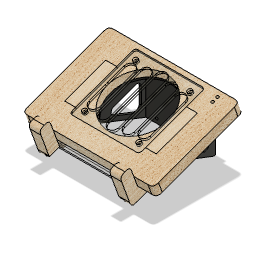
model_v2 (Autodesk Fusion 360 design; units mm, degrees)
Autodesk Fusion 360 part; units mm, degrees
note: some values were not read from the file. Set by a fixed rule: which face or edge a step refers to.
ref_plane "WorkPlane1" through (12.125, 0, 0) normal (0, -0.939693, -0.34202) x (1, 0, 0) in component "3dp"
sketch "Sketch1" plane through (12.125, 0, 0) normal (0, -0.939693, -0.34202) x (1, 0, 0) in component "3dp"
  line L0 (-87.125, 0) -> (62.875, 0)
  line L1 (62.875, 0) -> (62.875, 170)
  line L2 (62.875, 170) -> (-87.125, 170)
  line L3 (-87.125, 170) -> (-87.125, 0)
  line L4 (-12.125, 0) -> (-12.125, 170)
  line L5 (-87.125, 90) -> (62.875, 90) construction
  circle A0 centre (-12.125, 90) radius 70.05
  line L6 (-74.375, 27.75) -> (50.125, 27.75) construction
  line L7 (50.125, 27.75) -> (50.125, 152.25) construction
  line L8 (50.125, 152.25) -> (-74.375, 152.25) construction
  line L9 (-74.375, 152.25) -> (-74.375, 27.75) construction
  line L10 (-74.375, 27.75) -> (50.125, 152.25) construction
  line L11 (50.125, 27.75) -> (-74.375, 152.25) construction
  circle A1 centre (-74.375, 27.75) radius 2.25
  circle A2 centre (50.125, 27.75) radius 2.25
  circle A3 centre (50.125, 152.25) radius 2.25
  circle A4 centre (-74.375, 152.25) radius 2.25
  point P0 (-12.125, 90)
  point P1 (-12.125, 0)
  dimension "d2" = 150
  dimension "d3" = 170
  dimension "d4" = 90
  dimension "d5" = 140.1
  dimension "d6" = 124.5
  dimension "d7" = 124.5
  dimension "d8" = 4.5
  dimension "d9" = 4.5
  dimension "d10" = 4.5
  dimension "d11" = 4.5
  constraint horizontal L0
  constraint vertical L1
  constraint horizontal L2
  constraint vertical L3
  constraint midpoint L0 P1
  constraint midpoint L2 L4.end
  constraint coincident L3 L5.start
  constraint coincident L1 L5.end
  constraint perpendicular L1 L5
  constraint midpoint L5 P0
  constraint horizontal L6
  constraint perpendicular L6 L7
  constraint parallel L6 L8
  constraint parallel L7 L9
  constraint coincident L10 P0
  constraint coincident L11 P0
  constraint coincident P0 A0.centre
  constraint coincident L6.start L9.end
  constraint coincident L6.end L7.start
  constraint coincident L7.end L8.start
  constraint coincident L8.end L9.start
  constraint coincident P1 L4.start
  measures "d2" distance of L0.start L0.end
  measures "d3" distance of L0.start L2.end
  measures "d4" distance of L0 L5
  measures "d5" diameter of A0
  measures "d6" distance of L7.end L8.end
  measures "d7" distance of L6.end L7.end
  measures "d8" diameter of A1
  measures "d9" diameter of A2
  measures "d10" diameter of A3
  measures "d11" diameter of A4
extrude "Extrude1" add sketch "Sketch1" against normal blind 5 contours L0 L2 L3 L4 A0 | L0 L1 L2 L4 A0 makes body 1 in component "3dp"
sketch "Sketch2" plane through (0, 0, 0) normal (0, 0, 1) x (1, 0, 0) in component "3dp"
  line L0 (-75, 0) -> (75, 0)
  line L1 (75, 0) -> (75, -120)
  line L2 (75, -120) -> (-75, -120)
  line L3 (-75, -120) -> (-75, 0)
  line L4 (0, 0) -> (0, -120)
  line L5 (75, -60) -> (-75, -60)
  line L6 (-50, -10) -> (50, -10) construction
  line L7 (50, -10) -> (50, -110) construction
  line L8 (50, -110) -> (-50, -110) construction
  line L9 (-50, -110) -> (-50, -10) construction
  line L10 (-50, -10) -> (50, -110) construction
  line L11 (50, -10) -> (-50, -110) construction
  circle A0 centre (-50, -10) radius 3
  circle A1 centre (50, -10) radius 3
  circle A2 centre (-50, -110) radius 3
  circle A3 centre (50, -110) radius 3
  point P0 (0, -60)
  dimension "d14" = 120
  dimension "d15" = 150
  dimension "d16" = 100
  dimension "d17" = 100
  dimension "d18" = 6
  dimension "d19" = 6
  dimension "d20" = 6
  dimension "d21" = 6
  constraint horizontal L0
  constraint vertical L1
  constraint horizontal L2
  constraint vertical L3
  constraint midpoint L0 L4.start
  constraint midpoint L2 L4.end
  constraint midpoint L1 L5.start
  constraint midpoint L3 L5.end
  constraint coincident L4.start origin
  constraint horizontal L6
  constraint perpendicular L6 L7
  constraint parallel L6 L8
  constraint parallel L7 L9
  constraint coincident L10 P0
  constraint coincident L11 P0
  constraint midpoint L4 P0
  constraint coincident L6.start L9.end
  constraint coincident L6.end L7.start
  constraint coincident L8.end L9.start
  constraint coincident L7.end L8.start
  measures "d14" distance of L0.start L2.end
  measures "d15" distance of L0.start L0.end
  measures "d16" distance of L7.end L8.end
  measures "d17" distance of L6.end L7.end
  measures "d18" diameter of A0
  measures "d19" diameter of A1
  measures "d20" diameter of A2
  measures "d21" diameter of A3
extrude "Extrude2" add sketch "Sketch2" against normal blind 5 separate body makes body 2 in component "3dp"
sketch "Sketch3" plane through (75, 0, 0) normal (1, 0, 0) x (0, 0, -1) in component "3dp"
  line L0 (-161.4578, -53.445) -> (-1.7101, 4.6985)
  line L1 (5, 0) -> (5, -120)
  arc A0 (5, 0) -> (-2.5, 4.3301) centre (0, 0) ccw
  line L2 (0, 0) -> (-159.7477, -58.1434)
  line L3 (0, 0) -> (0, -120)
  line L4 (-159.7477, -58.1434) -> (0, -120)
  line L5 (-159.7477, -58.1434) -> (-161.4578, -53.445)
  line L6 (0, -120) -> (5, -120)
  constraint tangent L1 A0
  constraint tangent L0 A0
  constraint coincident L1.start A0.start
  constraint coincident L2.end L4.start
  constraint coincident L3.end L4.end
extrude "Extrude4" add sketch "Sketch3" along normal blind 5 bodies 1 2 in component "3dp"
extrude "Extrude6" add 1 faces at (75, 0.2452, -3.3152) along direction (-1, 0, 0) up to surface (150 mm away) on bodies 1 bodies 1 in component "3dp"
mirror "Mirror1" about plane through (0, 0, 0) normal (1, 0, 0) of "Extrude4" in component "3dp"
sketch "Sketch1 (2)" plane through (0, 4.6985, 1.7101) normal (0, 0.939693, 0.34202) x (1, 0, 0) in component "base"
  line L0 (80, 0) -> (-80, 0)
  line L1 (-150, 0) -> (150, 0)
  line L2 (150, 0) -> (150, -210)
  line L3 (150, -210) -> (-150, -210)
  line L4 (-150, -210) -> (-150, 0)
  line L5 (0, -210) -> (0, 0)
  dimension "d34" = 300
  dimension "d40" = 210
  constraint horizontal L1
  constraint vertical L2
  constraint horizontal L3
  constraint vertical L4
  constraint collinear L0 L1
  constraint midpoint L3 L5.start
  constraint midpoint L1 L5.end
  constraint coincident L5.end origin
  measures "d34" distance of L1.start L1.end
  measures "d40" distance of L1.start L3.end
extrude "Extrude1'" add sketch "Sketch1 (2)" along normal blind 25 separate body makes body 3 in component "base"
sketch "Sketch2 (2)" plane through (0, 4.6985, 1.7101) normal (0, -0.939693, -0.34202) x (-1, 0, 0) in component "base"
  line L0 (-150, -210) -> (150, -210)
  line L1 (150, -210) -> (150, 0)
  line L2 (150, 0) -> (-150, 0)
  line L3 (-150, 0) -> (-150, -210)
  circle A0 centre (0, -90) radius 70.05
  circle A1 centre (62.25, -27.75) radius 2.25
  circle A2 centre (62.25, -152.25) radius 2.25
  circle A3 centre (-62.25, -27.75) radius 2.25
  circle A4 centre (-62.25, -152.25) radius 2.25
  line L4 (-80, -170) -> (80, -170)
  line L5 (-80, -175) -> (80, -175) construction
  circle A5 centre (0, -175) radius 2.48
  dimension "d53" = 5
  dimension "d54" = 4.96
  constraint midpoint L5 A5.centre
  measures "d54" diameter of A5
extrude "Extrude2'" cut sketch "Sketch2 (2)" against normal up to surface (25 mm away) contours A0 | A1 | A2 | A3 | A4 bodies 3 in component "base"
sketch "Sketch3 (2)" plane through (0, 28.1908, 10.2606) normal (0, 0.939693, 0.34202) x (1, 0, 0) in component "base"
  circle A0 centre (-62.25, -152.25) radius 2.25
  circle A1 centre (0, -90) radius 70.05
  circle A2 centre (-62.25, -27.75) radius 2.25
  circle A3 centre (62.25, -152.25) radius 2.25
  circle A4 centre (62.25, -27.75) radius 2.25
  line L0 (-150, -210) -> (150, -210)
  line L1 (150, -210) -> (150, 0)
  line L2 (150, 0) -> (-150, 0)
  line L3 (-150, 0) -> (-150, -210)
  line L4 (80, -170) -> (-80, -170)
  line L5 (80, 0) -> (80, -170)
  line L6 (-80, 0) -> (-80, -170)
  line L7 (-74, -170) -> (74, -170)
  line L8 (80, -164) -> (80, -16)
  line L9 (74, -10) -> (-74, -10)
  line L10 (-80, -16) -> (-80, -164)
  arc A5 (-74, -10) -> (-80, -16) centre (-74, -16) ccw
  arc A6 (80, -16) -> (74, -10) centre (74, -16) ccw
  arc A7 (74, -170) -> (80, -164) centre (74, -164) ccw
  arc A8 (-80, -164) -> (-74, -170) centre (-74, -164) ccw
  point P0 (80, -170)
  point P1 (-80, -10)
  dimension "d46" = 6
  dimension "d47" = 6
  dimension "d48" = 6
  dimension "d49" = 6
  dimension "d116" = 160
  dimension "d117" = 160
  constraint horizontal L7
  constraint vertical L8
  constraint horizontal L9
  constraint vertical L10
  constraint coincident P1 L9
  constraint coincident P1 L10
  constraint tangent L9 A5
  constraint tangent L10 A5
  constraint tangent L8 A6
  constraint tangent L9 A6
  constraint coincident P0 L7
  constraint coincident P0 L8
  constraint tangent L7 A7
  constraint tangent L8 A7
  constraint tangent L10 A8
  constraint tangent L7 A8
  constraint collinear L4 L7
  constraint collinear L5 L8
  constraint collinear L6 L10
  measures "d46" radius of A5
  measures "d47" radius of A6
  measures "d48" radius of A7
  measures "d49" radius of A8
  measures "d116" distance of L8 L10
  measures "d117" distance of L7 L9
extrude "Extrude3" cut sketch "Sketch3 (2)" against normal blind 4.95 contours L4 L5 L6 L7 L8 L9 L10 A5 A6 A7 A8 bodies 3 in component "base"
sketch "Sketch1 (3)" plane through (80, 0, 0) normal (1, 0, 0) x (0, 0, -1) in component "legs"
  line L0 (-1.7101, 4.6985) -> (-161.4578, -53.445)
  line L1 (8.0022, -21.986) -> (-212.8255, -102.3607)
  line L2 (-1.7101, 4.6985) -> (8.0022, -21.986)
  line L3 (-161.4578, -53.445) -> (-159.7477, -58.1434)
  line L4 (-199.0456, -67.1258) -> (-207.5961, -43.6335)
  line L5 (-222.5379, -75.6763) -> (-231.0884, -52.184)
  line L6 (-222.5379, -75.6763) -> (-212.8255, -102.3607)
  line L7 (-207.5961, -43.6335) -> (-216.1466, -20.1411)
  line L8 (-216.1466, -20.1411) -> (-239.6389, -28.6916)
  line L9 (-239.6389, -28.6916) -> (-231.0884, -52.184)
  line L10 (-199.0456, -67.1258) -> (-161.4578, -53.445)
  line L11 (-207.5961, -43.6335) -> (-10.2606, 28.1908)
  line L12 (-108.9283, -7.7213) -> (-100.3778, -31.2137)
  line L13 (-108.9283, -7.7213) -> (-61.9437, 9.3797)
  line L14 (-61.9437, 9.3797) -> (-53.3932, -14.1126)
  line L15 (-108.9283, -7.7213) -> (-155.913, -24.8223)
  line L16 (-155.913, -24.8223) -> (-147.3625, -48.3147)
  dimension "d59" = 25
  dimension "d62" = 50
  dimension "d63" = 50
  constraint coincident L0.start L2.start
  constraint perpendicular L1 L2
  constraint parallel L5 L6
  constraint coincident L4.end L7.start
  constraint perpendicular L1 L7
  constraint perpendicular L5 L8
  constraint perpendicular L8 L9
  constraint coincident L4.start L10.start
  constraint coincident L0.end L3.start
  constraint midpoint L11 L12.start
  constraint coincident L0 L12.end
  constraint perpendicular L0 L12
  constraint perpendicular L12 L13
  constraint coincident L0 L14.end
  constraint perpendicular L0 L14
  constraint perpendicular L12 L15
  constraint coincident L0 L16.end
  constraint perpendicular L0 L16
  measures "d59" distance of L4.end L7.end
  measures "d62" distance of L12.start L13.end
  measures "d63" distance of L12.start L15.end
extrude "Extrude1''" add sketch "Sketch1 (3)" along normal blind 25 separate body contours L0 L1 L2 L4 L5 L6 L7 L8 L9 L10 | L0 L11 L12 L13 L14 | L0 L11 L12 L15 L16 makes body 4 in component "legs"
sketch "Sketch2 (3)" plane through (80, 0, 0) normal (-1, 0, 0) x (0, 0, 1) in component "legs"
  line L0 (155.913, -24.8223) -> (61.9437, 9.3797)
  line L1 (61.9437, 9.3797) -> (53.3932, -14.1126)
  line L2 (53.3932, -14.1126) -> (1.7101, 4.6985)
  line L3 (1.7101, 4.6985) -> (-8.0022, -21.986)
  line L4 (-8.0022, -21.986) -> (212.8255, -102.3607)
  line L5 (212.8255, -102.3607) -> (239.6389, -28.6916)
  line L6 (239.6389, -28.6916) -> (216.1466, -20.1411)
  line L7 (216.1466, -20.1411) -> (199.0456, -67.1258)
  line L8 (199.0456, -67.1258) -> (147.3625, -48.3147)
  line L9 (147.3625, -48.3147) -> (155.913, -24.8223)
  line L10 (199.0456, -67.1258) -> (189.3332, -93.8102)
  line L11 (194.3941, -65.4328) -> (184.6817, -92.1172)
  line L12 (-6.3092, -17.3345) -> (214.5185, -97.7092) construction
  line L13 (-4.6162, -12.683) -> (216.2115, -93.0578) construction
  line L14 (159.7477, -58.1434) -> (0, -120)
  line L15 (141.3408, -65.807) -> (216.2115, -93.0578)
  line L16 (141.3408, -65.807) -> (139.6478, -70.4585)
  line L17 (139.6478, -70.4585) -> (214.5185, -97.7092)
  dimension "d68" = 4.95
  dimension "d70" = -9.9
  dimension "d71" = 0.5
  constraint coincident L7.end L8.start
  constraint coincident L4 L10.end
  constraint perpendicular L4 L10
  constraint coincident L13 L15.start
  constraint parallel L12 L15
  constraint coincident L12 L16.end
  constraint perpendicular L12 L16
  constraint perpendicular L10 L17
  measures "d71" distance of L14 L15.start
extrude "Extrude2''" cut sketch "Sketch2 (3)" against normal blind 9.9 contours L8 L10 L11 L15 | L10 L11 L15 L17 | L11 L15 L16 L17 | L5 L10 L15 L17 | L4 L10 L11 L17 | L4 L5 L10 L17 bodies 4 in component "legs"
fillet "Fillet1" radius 12.5 tangency weight 2 4 edges at (92.5, -21.986, -8.0022) (92.5, -102.3607, 212.8255) (92.5, -28.6916, 239.6389) (92.5, -20.1411, 216.1466) on bodies 4 in component "legs"
mirror "Mirror1'" about plane through (0, 0, 0) normal (1, 0, 0) of bodies 4 makes body 5 in component "legs"
sketch "Sketch1 (4)" plane through (0, 23.5393, 8.5676) normal (0, 0.939693, 0.34202) x (1, 0, 0) in component "grill"
  circle A0 centre (62.25, -27.75) radius 2.25
  circle A1 centre (0, -90) radius 70.05
  circle A2 centre (62.25, -152.25) radius 2.25
  circle A3 centre (-62.25, -27.75) radius 2.25
  circle A4 centre (-62.25, -152.25) radius 2.25
  arc A5 (-80, -164) -> (-74, -170) centre (-74, -164) ccw
  line L0 (-74, -170) -> (74, -170)
  arc A6 (74, -170) -> (80, -164) centre (74, -164) ccw
  line L1 (80, -164) -> (80, -16)
  arc A7 (80, -16) -> (74, -10) centre (74, -16) ccw
  line L2 (74, -10) -> (-74, -10)
  arc A8 (-74, -10) -> (-80, -16) centre (-74, -16) ccw
  line L3 (-80, -16) -> (-80, -164)
  circle A9 centre (-62.25, -27.75) radius 5.25
  circle A10 centre (62.25, -27.75) radius 5.25
  circle A11 centre (-62.25, -152.25) radius 5.25
  circle A12 centre (62.25, -152.25) radius 5.25
  line L4 (0, -10) -> (0, -170)
  line L5 (-12, -32) -> (-12, -148)
  arc A13 (-12, -148) -> (12, -148) centre (0, -148) ccw
  line L6 (12, -148) -> (12, -32)
  arc A14 (12, -32) -> (-12, -32) centre (0, -32) ccw
  line L7 (0, -20) -> (0, -160) construction
  line L8 (-29, -20) -> (-29, -160) construction
  line L9 (-58, -20) -> (-58, -160) construction
  line L10 (-41, -39.7128) -> (-41, -140.2872)
  arc A15 (-41, -140.2872) -> (-17, -140.2872) centre (-29, -140.2872) ccw
  line L11 (-17, -140.2872) -> (-17, -39.7128)
  arc A16 (-17, -39.7128) -> (-41, -39.7128) centre (-29, -39.7128) ccw
  line L12 (-29, -27.7128) -> (-29, -152.2872) construction
  line L13 (-70, -47.4256) -> (-70, -132.5744)
  arc A17 (-70, -132.5744) -> (-46, -132.5744) centre (-58, -132.5744) ccw
  line L14 (-46, -132.5744) -> (-46, -47.4256)
  arc A18 (-46, -47.4256) -> (-70, -47.4256) centre (-58, -47.4256) ccw
  line L15 (-58, -35.4256) -> (-58, -144.5744) construction
  line L16 (0, -32) -> (-80, -53.2767) construction
  line L17 (-80, -90) -> (80, -90)
  line L18 (0, -148) -> (-80, -126.7233) construction
  line L19 (17, -140.2872) -> (17, -39.7128)
  arc A19 (41, -39.7128) -> (17, -39.7128) centre (29, -39.7128) ccw
  line L20 (41, -39.7128) -> (41, -140.2872)
  arc A20 (17, -140.2872) -> (41, -140.2872) centre (29, -140.2872) ccw
  arc A21 (46, -132.5744) -> (70, -132.5744) centre (58, -132.5744) ccw
  line L21 (46, -132.5744) -> (46, -47.4256)
  line L22 (70, -47.4256) -> (70, -132.5744)
  arc A22 (70, -47.4256) -> (46, -47.4256) centre (58, -47.4256) ccw
  line L23 (-70, -20) -> (-70, -160) construction
  line L24 (-70, -160) -> (70, -160) construction
  line L25 (70, -160) -> (70, -20) construction
  line L26 (70, -20) -> (-70, -20) construction
  dimension "d74" = 3
  dimension "d75" = 3
  dimension "d76" = 3
  dimension "d77" = 3
  dimension "d79" = -10
  dimension "d80" = 24
  dimension "d81" = 29
  dimension "d83" = 58
  dimension "d85" = 24
  dimension "d86" = 24
  constraint midpoint L2 L4.start
  constraint midpoint L0 L4.end
  constraint tangent L5 A13
  constraint tangent A13 L6
  constraint parallel L5 L6
  constraint tangent L6 A14
  constraint tangent L5 A14
  constraint midpoint A14 L7.start
  constraint midpoint A13 L7.end
  constraint midpoint L7.end L24
  constraint perpendicular L7 L24
  constraint midpoint L7.start L26
  constraint tangent L10 A15
  constraint tangent A15 L11
  constraint parallel L10 L11
  constraint tangent L11 A16
  constraint tangent L10 A16
  constraint midpoint A16 L12.start
  constraint midpoint A15 L12.end
  constraint coincident L8 L12.end
  constraint parallel L8 L12
  constraint tangent A1 A16
  constraint tangent A1 A15
  constraint tangent L13 A17
  constraint tangent A17 L14
  constraint parallel L13 L14
  constraint tangent L14 A18
  constraint tangent L13 A18
  constraint midpoint A18 L15.start
  constraint midpoint A17 L15.end
  constraint coincident L9 L15.end
  constraint parallel L9 L15
  constraint coincident A14.centre L16.start
  constraint coincident A16.centre L16
  constraint coincident A18.centre L16
  constraint coincident L3 L16.end
  constraint midpoint L3 L17.start
  constraint midpoint L1 L17.end
  constraint symmetric A14.centre L17 A13.centre
  constraint symmetric L16.end L17 L18.end
  constraint coincident A17.centre L18
  constraint symmetric L7 L10.start A19.start
  constraint symmetric L7 L10.end L20.end
  constraint symmetric L7 A15.end L19.start
  constraint symmetric L7 L11.end L19.end
  constraint symmetric L7 A15 A20
  constraint symmetric L7 A16 A19
  constraint symmetric L7 L13.start L22.start
  constraint symmetric L7 L13.end A21.end
  constraint symmetric L7 A17.end A21.start
  constraint symmetric L7 L14.end L21.end
  constraint symmetric L7 A17 A21
  constraint symmetric L7 A18 A22
  measures "d80" distance of L5 L6
  measures "d85" diameter of A15
  measures "d86" diameter of A17
extrude "Extrude1'''" add sketch "Sketch1 (4)" along normal up to surface (4.95 mm away) separate body contours A1 L0 A6 L1 L4 L17 A21 L22 | A1 L1 A7 L2 L4 L17 L22 A22 | A1 L17 A19 L20 L21 A22 | A1 L17 L20 A20 A21 L21 | A1 L4 L6 A14 L17 L19 A19 | A1 L4 A13 L6 L17 L19 A20 | A1 L4 L5 A14 L11 A16 L17 | A1 L2 A8 L3 L4 L13 A18 L17 | A1 A5 L0 L3 L4 L13 A17 L17 | A1 L4 L5 A13 A15 L11 L17 | A1 L10 A16 L14 A18 L17 | A1 L10 A15 A17 L14 L17 makes body 6 in component "grill"
sketch "Sketch1 (5)" plane through (0, -70.1312, 192.684) normal (0, -0.34202, 0.939693) x (1, 0, 0) in component "cover"
  line L0 (-80, -13.497) -> (-80, 5)
  line L1 (-80, 5) -> (-89.9, 5)
  line L2 (-89.9, 5) -> (-89.9, -13.497)
  line L3 (-89.9, -13.497) -> (-80, -13.497)
  line L4 (80, 5) -> (80, -13.497)
  line L5 (80, -13.497) -> (89.9, -13.497)
  line L6 (89.9, -13.497) -> (89.9, 5)
  line L7 (89.9, 5) -> (80, 5)
  line L8 (-89.9, 5) -> (89.9, 5)
  line L9 (89.9, 5) -> (89.9, -13.497)
  line L10 (89.9, -13.497) -> (-89.9, -13.497)
  line L11 (-89.9, -13.497) -> (-89.9, 5)
  line L12 (55, 5) -> (55, -13.497) construction
  circle A0 centre (55, -4.2485) radius 2.875
  dimension "d89" = 25
  dimension "d90" = 5.75
  constraint horizontal L8
  constraint vertical L9
  constraint horizontal L10
  constraint vertical L11
  constraint coincident L5.end L6.start
  constraint coincident L1.end L2.start
  constraint midpoint L12 A0.centre
  measures "d90" diameter of A0
extrude "Extrude1''''" add sketch "Sketch1 (5)" along normal blind 4.95 separate body makes body 7 in component "cover"
sketch "Sketch2 (4)" plane through (0, -12.683, -4.6162) normal (0, -0.939693, -0.34202) x (-1, 0, 0) in component "cover"
  line L0 (80, -155.3242) -> (80, -205.05)
  line L1 (80, -205.05) -> (89.9, -205.05)
  line L2 (89.9, -205.05) -> (89.9, -155.3242)
  line L3 (89.9, -155.3242) -> (80, -155.3242)
  line L4 (89.9, -205.05) -> (-89.9, -205.05)
  line L5 (-89.9, -205.05) -> (-89.9, -210)
  line L6 (-89.9, -210) -> (89.9, -210)
  line L7 (89.9, -210) -> (89.9, -205.05)
  line L8 (89.9, -155.3242) -> (-89.9, -155.3242)
  line L9 (-89.9, -155.3242) -> (-89.9, -210)
  line L10 (-89.9, -210) -> (89.9, -210)
  line L11 (89.9, -210) -> (89.9, -155.3242)
  constraint horizontal L8
  constraint vertical L9
  constraint horizontal L10
  constraint vertical L11
  constraint coincident L5.end L6.start
  constraint coincident L2.end L3.start
extrude "Extrude2'''" add sketch "Sketch2 (4)" along normal blind 4.95 separate body makes body 8 in component "cover"
combine "Combine1" operation cut target body 3 tool bodies 4 5 keep tools in component "base"
fillet "Fillet1'" radius 12.5 tangency weight 2 4 edges at (150, 16.4446, 5.9854) (-150, 16.4446, 5.9854) (-150, -55.3796, 203.3208) (150, -55.3796, 203.3208) on bodies 3 in component "base"
sketch "Sketch4" plane through (0, 4.6985, 1.7101) normal (0, -0.939693, -0.34202) x (-1, 0, 0) in component "base"
  line L0 (105, -55) -> (105, -155)
  line L1 (105, -155) -> (80, -155)
  line L2 (80, -155) -> (80, -55)
  line L3 (80, -55) -> (105, -55)
  circle A0 centre (62.25, -152.25) radius 2.25
  circle A1 centre (0, -90) radius 70.05
  circle A2 centre (62.25, -27.75) radius 2.25
  circle A3 centre (-62.25, -152.25) radius 2.25
  circle A4 centre (-62.25, -27.75) radius 2.25
  line L4 (-105, -155) -> (-105, -55)
  line L5 (-105, -55) -> (-80, -55)
  line L6 (-80, -55) -> (-80, -155)
  line L7 (-80, -155) -> (-105, -155)
  spline S0 degree 3 poles (-137.5, -210) (-139.8878, -210) (-142.1204, -209.8337) (-145.1029, -208.986) (-146.0407, -208.535) (-147.4853, -207.4182) (-148.0241, -206.7863) (-148.9372, -205.2061) (-149.2992, -204.1965) (-149.8776, -201.3864) (-150, -199.543) (-150, -197.5) knots 0 0 0 0 0.716343 0.716343 1.166029 1.166029 1.5643 1.5643 2.014339 2.014339 2.5976 2.5976 2.5976 2.5976
  line L8 (-137.5, -210) -> (137.5, -210)
  spline S1 degree 3 poles (150, -197.5) (150, -199.8878) (149.8337, -202.1204) (148.986, -205.1029) (148.535, -206.0407) (147.4182, -207.4853) (146.7863, -208.0241) (145.2061, -208.9372) (144.1965, -209.2992) (141.3864, -209.8776) (139.543, -210) (137.5, -210) knots 0 0 0 0 0.716343 0.716343 1.166029 1.166029 1.5643 1.5643 2.014339 2.014339 2.5976 2.5976 2.5976 2.5976
  line L9 (150, -197.5) -> (150, -12.5)
  spline S2 degree 3 poles (137.5, 0) (139.8878, 0) (142.1204, -0.1663) (145.1029, -1.014) (146.0407, -1.465) (147.4853, -2.5818) (148.0241, -3.2137) (148.9372, -4.7939) (149.2992, -5.8035) (149.8776, -8.6136) (150, -10.457) (150, -12.5) knots 0 0 0 0 0.716343 0.716343 1.166029 1.166029 1.5643 1.5643 2.014339 2.014339 2.5976 2.5976 2.5976 2.5976
  line L10 (137.5, 0) -> (-137.5, 0)
  spline S3 degree 3 poles (-150, -12.5) (-150, -10.1122) (-149.8337, -7.8796) (-148.986, -4.8971) (-148.535, -3.9593) (-147.4182, -2.5147) (-146.7863, -1.9759) (-145.2061, -1.0628) (-144.1965, -0.7008) (-141.3864, -0.1224) (-139.543, 0) (-137.5, 0) knots 0 0 0 0 0.716343 0.716343 1.166029 1.166029 1.5643 1.5643 2.014339 2.014339 2.5976 2.5976 2.5976 2.5976
  line L11 (-150, -12.5) -> (-150, -197.5)
  line L12 (-105, 0) -> (-105, -55)
  circle A5 centre (-111, -12) radius 3
  circle A6 centre (-111, -24) radius 3
  dimension "d103" = 6
  dimension "d104" = 12
  dimension "d105" = 6
  dimension "d118" = 6
  dimension "d119" = 12
  dimension "d120" = 6
  measures "d103" diameter of A5
  measures "d104" distance of L10 A5.centre
  measures "d105" distance of L12 A5.centre
  measures "d118" diameter of A6
  measures "d119" vertical distance of A5.centre A6.centre
  measures "d120" distance of L12 A6.centre
extrude "Extrude4'" cut sketch "Sketch4" against normal up to surface (25 mm away) contours A5 | A6 bodies 3 in component "base"
sketch "Sketch4 (2)" plane through (-80, 0, 0) normal (1, 0, 0) x (0, 0, -1) in component "legs"
  spline S0 degree 3 poles (-3.7439, -26.2612) (-1.5001, -25.4446) (0.541, -24.5247) (3.0536, -22.708) (3.7806, -21.9635) (4.7562, -20.42) (5.0464, -19.6419) (5.3639, -17.8447) (5.3588, -16.7722) (4.9412, -13.9337) (4.4257, -12.1596) (3.727, -10.2398) knots 0 0 0 0 0.716343 0.716343 1.166029 1.166029 1.5643 1.5643 2.014339 2.014339 2.5976 2.5976 2.5976 2.5976
  line L0 (3.727, -10.2398) -> (-1.7101, 4.6985)
  line L1 (-1.7101, 4.6985) -> (-53.3932, -14.1126)
  line L2 (-53.3932, -14.1126) -> (-61.9437, 9.3797)
  line L3 (-61.9437, 9.3797) -> (-155.913, -24.8223)
  line L4 (-155.913, -24.8223) -> (-147.3625, -48.3147)
  line L5 (-147.3625, -48.3147) -> (-194.3941, -65.4328)
  line L6 (-194.3941, -65.4328) -> (-188.0677, -82.8143)
  line L7 (-188.0677, -82.8143) -> (-141.3408, -65.807)
  line L8 (-141.3408, -65.807) -> (-139.6478, -70.4585)
  line L9 (-139.6478, -70.4585) -> (-186.3747, -87.4657)
  line L10 (-186.3747, -87.4657) -> (-184.6817, -92.1172)
  line L11 (-184.6817, -92.1172) -> (-3.7439, -26.2612)
  line L12 (-161.4578, -53.445) -> (-159.7477, -58.1434)
  line L13 (-179.312, -59.9433) -> (-167.096, -55.4971)
  line L14 (-167.096, -55.4971) -> (-165.0439, -61.1352)
  line L15 (-165.0439, -61.1352) -> (-177.2599, -65.5815)
  line L16 (-179.312, -59.9433) -> (-177.2599, -65.5815)
  dimension "d108" = 6
  dimension "d109" = 13
  dimension "d110" = 6
  constraint parallel L5 L13
  constraint perpendicular L13 L14
  constraint perpendicular L14 L15
  constraint perpendicular L13 L16
  constraint collinear L5 L13
  measures "d108" distance of L13.start L15.end
  measures "d109" distance of L14.end L15.end
  measures "d110" distance of L12 L14
extrude "Extrude4''" cut sketch "Sketch4 (2)" against normal up to surface (25 mm away) contours L5 L13 L14 L15 L16 bodies 5 in component "legs"
sketch "Sketch9" plane through (75, 0, 0) normal (-1, 0, 0) x (0, 0, 1) in component "3dp"
  line L0 (159.7477, -58.1434) -> (0, 0)
  line L1 (0, 0) -> (0, -120)
  line L2 (0, -120) -> (159.7477, -58.1434)
  line L3 (3.7439, -26.2612) -> (184.6817, -92.1172)
  line L4 (23.4202, -44.0646) -> (73.1379, -62.1604)
  line L5 (23.6109, -100.134) -> (73.3286, -80.8826)
  line L6 (10, -53.4615) -> (10, -90.8087)
  arc A0 (23.4202, -44.0646) -> (10, -53.4615) centre (20, -53.4615) ccw
  arc A1 (10, -90.8087) -> (23.6109, -100.134) centre (20, -90.8087) ccw
  arc A2 (73.3286, -80.8826) -> (73.1379, -62.1604) centre (69.7177, -71.5573) ccw
  dimension "d134" = 10
  dimension "d135" = 10
  dimension "d136" = 10
  dimension "d137" = 10
  dimension "d138" = 10
  constraint tangent L4 A0
  constraint tangent L6 A0
  constraint tangent L6 A1
  constraint tangent L5 A1
  constraint tangent L4 A2
  constraint tangent L5 A2
  measures "d134" distance of L2 L5
  measures "d135" distance of L1 L6
  measures "d136" radius of A0
  measures "d137" radius of A1
  measures "d138" radius of A2
extrude "Extrude9" cut sketch "Sketch9" along normal up to surface (155 mm away) and the other way up to surface (5 mm away) contours L4 L5 L6 A0 A1 A2 bodies 1 in component "3dp"
sketch "Sketch8" plane through (0, 0, 0) normal (0, -0.939693, -0.34202) x (-1, 0, 0) in component "3dp"
  circle A0 centre (-62.25, -27.75) radius 2.25
  circle A1 centre (-62.25, -152.25) radius 2.25
  circle A2 centre (62.25, -152.25) radius 2.25
  circle A3 centre (62.25, -27.75) radius 2.25
  circle A4 centre (0, -90) radius 70.05
  line L0 (75, -170) -> (75, 0)
  line L1 (75, 0) -> (-75, 0)
  line L2 (-75, 0) -> (-75, -170)
  line L3 (-75, -170) -> (75, -170)
sketch "Sketch5" plane through (80, 0, 0) normal (-1, 0, 0) x (0, 0, 1) in component "legs"
  spline S0 degree 3 poles (3.7439, -26.2612) (1.5001, -25.4446) (-0.541, -24.5247) (-3.0536, -22.708) (-3.7806, -21.9635) (-4.7562, -20.42) (-5.0464, -19.6419) (-5.3639, -17.8447) (-5.3588, -16.7722) (-4.9412, -13.9337) (-4.4257, -12.1596) (-3.727, -10.2398) knots 0 0 0 0 0.716343 0.716343 1.166029 1.166029 1.5643 1.5643 2.014339 2.014339 2.5976 2.5976 2.5976 2.5976
  line L0 (3.7439, -26.2612) -> (184.6817, -92.1172)
  line L1 (184.6817, -92.1172) -> (186.3747, -87.4657)
  line L2 (188.0677, -82.8143) -> (194.3941, -65.4328)
  line L3 (194.3941, -65.4328) -> (147.3625, -48.3147)
  line L4 (147.3625, -48.3147) -> (155.913, -24.8223)
  line L5 (155.913, -24.8223) -> (61.9437, 9.3797)
  line L6 (61.9437, 9.3797) -> (53.3932, -14.1126)
  line L7 (53.3932, -14.1126) -> (1.7101, 4.6985)
  line L8 (1.7101, 4.6985) -> (-3.727, -10.2398)
  line L9 (27.0818, -4.5361) -> (21.4436, -2.484)
  circle A0 centre (23.2367, -6.3291) radius 3
  line L10 (21.4436, -2.484) -> (20.4176, -5.303)
  line L11 (27.0818, -4.5361) -> (26.0557, -7.3552)
  circle A1 centre (163.2509, -57.2901) radius 3
  line L12 (22.2106, -9.1482) -> (162.2248, -60.1092)
  line L13 (164.2769, -54.471) -> (27.0818, -4.5361)
  line L14 (161.4578, -53.445) -> (159.7477, -58.1434)
  line L15 (166.0699, -58.3162) -> (167.096, -55.4971)
  line L16 (167.096, -55.4971) -> (164.2769, -54.471)
  dimension "d123" = 6
  dimension "d124" = 6
  constraint coincident L9.end L10.start
  constraint perpendicular L7 L10
  constraint coincident L9.start L11.start
  constraint perpendicular L7 L11
  constraint tangent L9 A0
  constraint tangent A0 L11
  constraint coincident A0 L11.end
  constraint coincident A0 L10.end
  constraint tangent L3 A1
  constraint tangent A1 L12
  constraint tangent A0 L12
  constraint coincident A0 L12.start
  constraint coincident A1 L12.end
  constraint coincident L3 L13.start
  constraint coincident A1 L13.start
  constraint tangent A1 L14
  constraint coincident L3 L15.end
  constraint perpendicular L3 L15
  constraint tangent A1 L15
  constraint coincident A1 L15.start
  measures "d123" diameter of A0
  measures "d124" diameter of A1
extrude "Extrude5" [rolled back] along distance -9.9 taper angle 0 in component "legs"
sketch "Sketch7" plane through (105, 0, 0) normal (1, 0, 0) x (0, 0, -1) in component "legs"
  spline S0 degree 3 poles (-227.8927, -24.4164) (-225.6489, -23.5997) (-223.4941, -22.9924) (-220.4015, -22.7689) (-219.366, -22.872) (-217.6266, -23.4273) (-216.9041, -23.8368) (-215.5056, -25.0094) (-214.8202, -25.8343) (-213.3156, -28.2772) (-212.5701, -29.9675) (-211.8713, -31.8873) knots 0 0 0 0 0.716343 0.716343 1.166029 1.166029 1.5643 1.5643 2.014339 2.014339 2.5976 2.5976 2.5976 2.5976
  spline S1 degree 3 poles (-235.3636, -40.4378) (-236.1803, -38.194) (-236.7876, -36.0391) (-237.0111, -32.9466) (-236.908, -31.9111) (-236.3527, -30.1717) (-235.9432, -29.4492) (-234.7706, -28.0507) (-233.9457, -27.3653) (-231.5028, -25.8607) (-229.8125, -25.1151) (-227.8927, -24.4164) knots 0 0 0 0 0.716343 0.716343 1.166029 1.166029 1.5643 1.5643 2.014339 2.014339 2.5976 2.5976 2.5976 2.5976
  line L0 (-235.3636, -40.4378) -> (-217.1008, -90.6146)
  spline S2 degree 3 poles (-201.0794, -98.0855) (-203.3232, -98.9022) (-205.478, -99.5094) (-208.5705, -99.7329) (-209.6061, -99.6299) (-211.3455, -99.0745) (-212.0679, -98.665) (-213.4664, -97.4924) (-214.1519, -96.6676) (-215.6565, -94.2247) (-216.402, -92.5344) (-217.1008, -90.6146) knots 0 0 0 0 0.716343 0.716343 1.166029 1.166029 1.5643 1.5643 2.014339 2.014339 2.5976 2.5976 2.5976 2.5976
  line L1 (-201.0794, -98.0855) -> (-3.7439, -26.2612)
  spline S3 degree 3 poles (3.727, -10.2398) (4.5437, -12.4836) (5.151, -14.6385) (5.3744, -17.731) (5.2714, -18.7665) (4.716, -20.506) (4.3066, -21.2284) (3.134, -22.6269) (2.3091, -23.3123) (-0.1338, -24.817) (-1.8241, -25.5625) (-3.7439, -26.2612) knots 0 0 0 0 0.716343 0.716343 1.166029 1.166029 1.5643 1.5643 2.014339 2.014339 2.5976 2.5976 2.5976 2.5976
  line L2 (3.727, -10.2398) -> (-1.7101, 4.6985)
  line L3 (-1.7101, 4.6985) -> (-53.3932, -14.1126)
  line L4 (-53.3932, -14.1126) -> (-61.9437, 9.3797)
  line L5 (-61.9437, 9.3797) -> (-155.913, -24.8223)
  line L6 (-155.913, -24.8223) -> (-147.3625, -48.3147)
  line L7 (-147.3625, -48.3147) -> (-199.0456, -67.1258)
  line L8 (-199.0456, -67.1258) -> (-211.8713, -31.8873)
  line L9 (-53.3932, -14.1126) -> (-21.4436, -2.484)
  line L10 (-21.4436, -2.484) -> (-20.4176, -5.303)
  arc A0 (-22.2106, -9.1482) -> (-20.4176, -5.303) centre (-23.2367, -6.3291) ccw
  line L11 (-22.2106, -9.1482) -> (-162.2248, -60.1092)
  arc A1 (-166.0699, -58.3162) -> (-162.2248, -60.1092) centre (-163.2509, -57.2901) ccw
  line L12 (-167.096, -55.4971) -> (-147.3625, -48.3147)
  line L13 (-147.3625, -48.3147) -> (-53.3932, -14.1126)
  circle A2 centre (-23.2367, -6.3291) radius 3
  line L14 (-27.0818, -4.5361) -> (-26.0557, -7.3552)
  line L15 (-166.0699, -58.3162) -> (-167.096, -55.4971)
  dimension "d128" = 6
  constraint concentric A0 A2
  constraint coincident L3 L14.start
  constraint perpendicular L3 L14
  constraint tangent A2 L14
  constraint coincident A2 L14.end
  measures "d128" diameter of A2
extrude "Extrude6'" [rolled back] side1offset 0 taper angle 0 in component "legs"
component "3dp" placed x (1, 0, 0) y (0, 1, 0) z (0, 0, 1) at (0, 0, 0)
component "base" placed x (1, 0, 0) y (0, 1, 0) z (0, 0, 1) at (0, 0, 0)
component "legs" placed x (1, 0, 0) y (0, 1, 0) z (0, 0, 1) at (0, 0, 0)
component "grill" placed x (1, 0, 0) y (0, 1, 0) z (0, 0, 1) at (0, 0, 0)
component "cover" placed x (1, 0, 0) y (0, 1, 0) z (0, 0, 1) at (0, 0, 0)
equation "d2 = 140 mm + 10 mm"
equation "d4 = 20 mm + ( 140 / 2 ) * 1 mm"
equation "d7 = d6"
equation "d9 = d8"
equation "d10 = d8"
equation "d11 = d8"
equation "d15 = d2"
equation "d17 = d16"
equation "wdthick = 25 mm"
equation "d36 = wdthick"
equation "laserthick = 4.95 mm"
equation "d51 = -laserthick"
equation "d57 = -wdthick"
equation "d59 = wdthick"
equation "d64 = wdthick"
equation "d68 = laserthick"
equation "d69 = -laserthick"
equation "d70 = -laserthick * 2"
equation "d72 = -laserthick * 2"
equation "d75 = d74"
equation "d76 = d74"
equation "d77 = d74"
equation "d81 = d80 + 5 mm"
equation "d83 = d81 * 2"
equation "d89 = wdthick"
equation "d91 = laserthick"
equation "d93 = laserthick"
equation "d96 = wdthick / 2"
equation "d98 = wdthick / 2"
equation "d104 = ( 6 * 2 ) * 1 mm"
equation "d117 = d116"
equation "d119 = d104"
equation "d120 = d105"
equation "d125 = -laserthick * 2"
